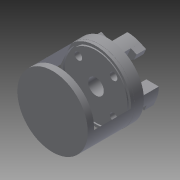
# Autodesk Inventor part: bayonet container
Saved by Autodesk Inventor 2015 (Build 190159000, 159)
## iProperties
Created: 2014-06-10
Part Number: bayonet container
Material: Generic
Document SubType Name: Modeling
Designer: ericd_000
Density: 1 g/cm^3
Appearance: Default
Author: ericd_000
Autodesk Inventor part; units mm, degrees
ref_plane "YZ Plane" through (0, 0, 0) normal (1, 0, 0) x (0, 1, 0)
ref_plane "XZ Plane" through (0, 0, 0) normal (0, 1, 0) x (-1, 0, 0)
ref_plane "XY Plane" through (0, 0, 0) normal (0, 0, 1) x (1, 0, 0)
sketch "Sketch1" plane through (0, 0, 0) normal (0, 1, 0) x (-1, 0, 0)
  circle A0 centre (0, 0) radius 25
  circle A1 centre (0, 0) radius 5.5
  circle A2 centre (14, 14) radius 3
  circle A3 centre (-14, 14) radius 3
  circle A4 centre (-14, -14) radius 3
  circle A5 centre (14, -14) radius 3
  line L0 (14, 14) -> (14, -14) construction
  line L1 (14, -14) -> (-14, -14) construction
  circle A6 centre (0, 0) radius 15
  point P0 (14, 0)
  point P1 (0, -14)
  dimension "d0" = 50
  dimension "d1" = 11
  dimension "d2" = 6
  dimension "d3" = 6
  dimension "d4" = 6
  dimension "d5" = 6
  dimension "d6" = 28
  dimension "d7" = 28
  dimension "d8" = 28
  dimension "d9" = 28
  dimension "d10" = 30
  constraints: 7 centre point, 4 end point, 3 coincident, 2 midpoint, 1 horizontal, 1 horizontal alignment, 1 vertical, 1 vertical alignment
  measures "d0" diameter of A0
  measures "d1" diameter of A1
  measures "d2" diameter of A2
  measures "d3" diameter of A5
  measures "d4" diameter of A4
  measures "d5" diameter of A3
  measures "d6" distance of L0.end L0.start
  measures "d7" distance of A3.centre L0.start
  measures "d8" distance of L1.end A3.centre
  measures "d9" distance of L0.end L1.end
  measures "d10" diameter of A6
extrude "Extrusion1" add sketch "Sketch1" along normal blind 5 contours A0
sketch "Sketch2" plane through (0, 5, 0) normal (0, 1, 0) x (1, 0, 0)
  circle A0 centre (0, 0) radius 25
  circle A1 centre (0, 0) radius 15
  constraints: 2 centre point, 2 coincident
sketch "Sketch3" plane through (0, 5, 0) normal (0, 1, 0) x (1, 0, 0)
  circle A0 centre (0, 0) radius 15 projected
  line L0 (-13.6716, -6.1716) -> (-22.4177, -10.1197)
  circle A1 centre (0, 0) radius 15 projected
  line L1 (6.1716, -13.6716) -> (10.1545, -22.4948)
  line L2 (-6.1716, 13.6716) -> (-10.3269, 22.8767)
  line L3 (13.6716, 6.1716) -> (22.7088, 10.2511)
  circle A2 centre (-14, -14) radius 3 projected
  circle A3 centre (14, -14) radius 3 projected
  circle A4 centre (14, 14) radius 3 projected
  circle A5 centre (-14, 14) radius 3 projected
  circle A6 centre (0, 0) radius 25 projected
  dimension "d14" = 7
  dimension "d15" = 7
  dimension "d16" = 7
  dimension "d17" = 7
  constraints: 8 end point, 7 point on circle, 3 line through centre, 1 collinear
  measures "d14" distance from line of L0 A2.centre
  measures "d15" distance from line of L1 A3.centre
  measures "d16" distance from line of L3 A4.centre
  measures "d17" distance from line of L2 A5.centre
extrude "Extrusion2" add sketch "Sketch3" along normal blind 20
sketch "Sketch4" plane through (0, 25, 0) normal (0, 1, 0) x (1, 0, 0)
  line L0 (6.1716, -13.6716) -> (10.2859, -22.7859)
  line L1 (25, 0) -> (15, 0)
  circle A0 centre (14, -14) radius 3 projected
  arc A1 (6.1716, -13.6716) -> (15, 0) centre (0, 0) ccw
  arc A2 (10.2859, -22.7859) -> (25, 0) centre (0, 0) ccw
  line L2 (-13.6716, -6.1716) -> (-22.7859, -10.2859)
  circle A3 centre (0, 0) radius 15 projected
  line L3 (-6.1716, 13.6716) -> (-10.2859, 22.7859)
  line L4 (13.6716, 6.1716) -> (22.7859, 10.2859)
  circle A4 centre (-14, -14) radius 3 projected
  circle A5 centre (-14, 14) radius 3 projected
  circle A6 centre (14, 14) radius 3 projected
  line L5 (-0.0013, -15) -> (-0.0021, -25)
  line L6 (-15, 0.0013) -> (-25, 0.0021)
  line L7 (0.0021, 25) -> (0.0013, 15)
  arc A7 (-0.0021, -25) -> (10.2859, -22.7859) centre (0, 0) ccw
  arc A8 (-0.0013, -15) -> (6.1716, -13.6716) centre (0, 0) ccw
  arc A9 (-13.6716, -6.1716) -> (-0.0013, -15) centre (0, 0) ccw
  arc A10 (-22.7859, -10.2859) -> (-0.0021, -25) centre (0, 0) ccw
  arc A11 (-25, 0.0021) -> (-22.7859, -10.2859) centre (0, 0) ccw
  arc A12 (-15, 0.0013) -> (-13.6716, -6.1716) centre (0, 0) ccw
  arc A13 (-10.2859, 22.7859) -> (-25, 0.0021) centre (0, 0) ccw
  arc A14 (-6.1716, 13.6716) -> (-15, 0.0013) centre (0, 0) ccw
  arc A15 (0.0013, 15) -> (-6.1716, 13.6716) centre (0, 0) ccw
  arc A16 (0.0021, 25) -> (-10.2859, 22.7859) centre (0, 0) ccw
  arc A17 (22.7859, 10.2859) -> (0.0021, 25) centre (0, 0) ccw
  arc A18 (13.6716, 6.1716) -> (0.0013, 15) centre (0, 0) ccw
  arc A19 (15, 0) -> (13.6716, 6.1716) centre (0, 0) ccw
  arc A20 (25, 0) -> (22.7859, 10.2859) centre (0, 0) ccw
  arc A21 (-0.0021, -25) -> (10.2859, -22.7859) centre (0, 0) ccw
  arc A22 (15, 0) -> (13.6716, 6.1716) centre (0, 0) ccw
  arc A23 (-13.6716, -6.1716) -> (-0.0013, -15) centre (0, 0) ccw
  arc A24 (-0.0013, -15) -> (6.1716, -13.6716) centre (0, 0) ccw
  dimension "d21" = 7
  dimension "d24" = 7
  dimension "d25" = 7
  dimension "d26" = 7
  dimension "d27" = 65.705
  dimension "d28" = 65.7
  dimension "d29" = 65.7
  dimension "d30" = 65.7
  constraints: 45 point on circle, 20 centre point, 16 end point, 9 concentric, 1 collinear, 1 horizontal
  measures "d21" distance from line of L0 A0.centre
  measures "d24" distance from line of L2 A4.centre
  measures "d25" distance from line of A5.centre L3
  measures "d26" distance from line of L4 A6.centre
  measures "d27" angle of L1 L0
  measures "d28" angle of L7 L4
  measures "d29" angle of L6 L3
  measures "d30" angle of L5 L2
extrude "Extrusion4" cut sketch "Sketch4" against normal blind 15 contours A1 L1 A2 L0 | L5 A10 L2 A3 | A3 L7 A17 L4 | L6 A13 L3 A3
sketch "Sketch5" plane through (10.2859, 10, 22.7859) normal (0.9114378, 0, -0.4114378) x (-0.4114378, 0, -0.9114378)
  line L0 (10, 15) -> (10, 0) projected
  line L1 (0.0055, 15) -> (10, 15)
  line L2 (10, 15) -> (10, 7.5)
  line L3 (10, 7.5) -> (0.0055, 7.5)
  line L4 (0.0055, 7.5) -> (0.0055, 15)
  point P0 (25, -10)
  dimension "d33" = 7.5
  constraints: 8 end point, 2 parallel, 1 horizontal, 1 midpoint, 1 perpendicular
  measures "d33" distance of L3.end L1.start
sketch "Sketch6" plane through (22.7859, 10, -10.2859) normal (-0.4114378, 0, -0.9114378) x (-0.9114378, 0, 0.4114378)
  line L0 (10, 15) -> (10, 0) projected
  line L1 (10, 7.5) -> (0, 7.5)
  line L2 (0, 7.5) -> (0, 15)
  line L3 (0, 15) -> (10, 15)
  line L4 (10, 15) -> (10, 7.5)
  point P0 (25, -10)
  dimension "d34" = 7.5
  constraints: 8 end point, 2 parallel, 1 horizontal, 1 midpoint, 1 perpendicular
  measures "d34" distance of L1.end L2.end
sketch "Sketch7" plane through (-10.2859, 10, -22.7859) normal (-0.9114378, 0, 0.4114378) x (0.4114378, 0, 0.9114378)
  line L0 (10, 15) -> (10, 0) projected
  line L1 (0, 15) -> (10, 15)
  line L2 (10, 15) -> (10, 7.5)
  line L3 (10, 7.5) -> (0, 7.5)
  line L4 (0, 7.5) -> (0, 15)
  point P0 (25, -10)
  dimension "d35" = 7.5
  constraints: 8 end point, 2 parallel, 1 horizontal, 1 midpoint, 1 perpendicular
  measures "d35" distance of L3.end L1.start
sketch "Sketch8" plane through (-22.7859, 10, 10.2859) normal (0.4114378, 0, 0.9114378) x (0.9114378, 0, -0.4114378)
  line L0 (10, 15) -> (10, 0) projected
  line L1 (0, 15) -> (10, 15)
  line L2 (10, 15) -> (10, 7.5)
  line L3 (10, 7.5) -> (0, 7.5)
  line L4 (0, 7.5) -> (0, 15)
  point P0 (25, -10)
  dimension "d36" = 7.5
  constraints: 8 end point, 2 parallel, 1 horizontal, 1 midpoint, 1 perpendicular
  measures "d36" distance of L3.end L1.start
extrude "Extrusion5" add sketch "Sketch5" along normal blind 5
extrude "Extrusion6" add sketch "Sketch6" along normal blind 5
extrude "Extrusion7" add sketch "Sketch7" along normal blind 5
extrude "Extrusion8" add sketch "Sketch8" along normal blind 5
sketch "Sketch9" plane through (0, 0, 0) normal (0, -1, 0) x (1, 0, 0)
  circle A0 centre (0, 0) radius 6.25
  circle A1 centre (0, 0) radius 15
  dimension "d45" = 12.5
  dimension "d48" = 30
  constraints: 2 centre point, 2 coincident
  measures "d45" diameter of A0
  measures "d48" diameter of A1
extrude "Extrusion9" add sketch "Sketch9" against normal blind 10
sketch "Sketch11" plane through (0, 25, 0) normal (0, 1, 0) x (1, 0, 0)
  line L0 (6.1716, -13.6716) -> (10.7288, -11.6144) projected
  line L1 (7.5288, -13.0589) -> (12.7848, -16.1691)
  line L2 (10.7288, -11.6144) -> (14.8409, -20.7237) projected
  point P0 (0, 0)
  dimension "d53" = 3.2
  constraints: 2 end point, 1 midpoint, 1 point on line
  measures "d53" horizontal distance of L0.end L1.start
extrude "Extrusion11" cut sketch "Sketch11" against normal up to next
sketch "Sketch12" plane through (0, 25, 0) normal (0, 1, 0) x (1, 0, 0)
  line L0 (-10.7288, 11.6144) -> (-14.8431, 20.7288) projected
  line L1 (-12.7859, 16.1716) -> (-7.5288, 13.0589)
  line L2 (-6.1716, 13.6716) -> (-10.7288, 11.6144) projected
  point P0 (0, 0)
  dimension "d60" = 3.2
  constraints: 2 end point, 1 midpoint, 1 point on line
  measures "d60" horizontal distance of L0.start L1.end
extrude "Extrusion12" cut sketch "Sketch12" against normal up to next
sketch "Sketch13" plane through (0, 25, 0) normal (0, 1, 0) x (1, 0, 0)
  line L0 (-11.6144, -10.7288) -> (-20.7288, -14.8431) projected
  line L1 (-16.1716, -12.7859) -> (-13.0589, -7.5288)
  line L2 (-13.6716, -6.1716) -> (-11.6144, -10.7288) projected
  point P0 (0, 0)
  dimension "d61" = 3.2
  constraints: 2 end point, 1 midpoint, 1 point on line
  measures "d61" vertical distance of L0.start L1.end
extrude "Extrusion13" cut sketch "Sketch13" against normal up to next
sketch "Sketch14" plane through (0, 0, 0) normal (0, -1, 0) x (1, 0, 0)
  circle A0 centre (0, 0) radius 28
  circle A1 centre (0, 0) radius 26
  dimension "d64" = 56
  dimension "d65" = 52
  constraints: 2 centre point, 1 coincident
  measures "d64" diameter of A0
  measures "d65" diameter of A1
extrude "Extrusion14" add sketch "Sketch14" along normal mid plane 5
sketch "Sketch16" plane through (0, 2.5, 0) normal (0, 1, 0) x (1, 0, 0)
  circle A0 centre (0, 0) radius 25
  circle A1 centre (0, 0) radius 28.1055
  constraints: 2 centre point, 2 coincident
extrude "Extrusion17" add sketch "Sketch16" along normal up to surface (7.5 mm away)
sketch "Sketch17" plane through (0, -2.5, 0) normal (0, -1, 0) x (1, 0, 0)
  circle A0 centre (0, 0) radius 26
  circle A1 centre (0, 0) radius 28
  dimension "d74" = 52
  dimension "d75" = 56
  constraints: 2 centre point, 2 coincident
  measures "d74" diameter of A0
  measures "d75" diameter of A1
extrude "Extrusion18" add sketch "Sketch17" along normal blind 27
ref_plane "Work Plane1" through (11.5203, 0, 25.5203) normal (0.4114378, 0, 0.9114378) x (0, 1, 0)
sketch "Sketch18" plane through (11.5203, 0, 25.5203) normal (0.4114378, 0, 0.9114378) x (0, 1, 0)
  line L0 (0, -6.25) -> (0, 6.25) projected
  line L1 (-29.5, 28) -> (-29.5, -28) projected
  line L2 (0, 26) -> (-29.5, 26)
  line L3 (-29.5, 26) -> (-29.5, -26)
  line L4 (-29.5, -26) -> (0, -26)
  line L5 (0, -26) -> (0, 26)
  point P0 (0, 0)
  dimension "d80" = 52
  dimension "d81" = 26
  constraints: 8 end point, 2 parallel, 2 point on line, 1 horizontal, 1 perpendicular
  measures "d80" distance of L4.end L2.start
  measures "d81" distance from line of L4 point (0, 0)
extrude "Extrusion19" cut sketch "Sketch18" against normal through all
sketch "Sketch19" plane through (0, -29.5, 0) normal (0, -1, 0) x (1, 0, 0)
  circle A0 centre (0, 0) radius 28
  dimension "d82" = 56
  constraints: 1 centre point, 1 coincident
  measures "d82" diameter of A0
extrude "Extrusion20" add sketch "Sketch19" along normal blind 5
sketch "Sketch20" plane through (0, -29.5, 0) normal (0, 1, 0) x (1, 0, 0)
  circle A0 centre (0, 0) radius 4.2
  dimension "d85" = 8.4
  constraints: 1 centre point, 1 coincident
  measures "d85" diameter of A0
extrude "Extrusion21" add sketch "Sketch20" along normal blind 5
body "Solid1"
